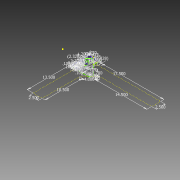
# Autodesk Inventor part: Phone_Holder
Saved by Autodesk Inventor 2013 (Build 170138000, 138)
## iProperties
Created: 2015-03-29
Part Number: Phone_Holder
Material: Generic
Document SubType Name: Modeling
Designer: Pat
Density: 1 g/cm^3
Author: Pat
Autodesk Inventor part; units mm, degrees
ref_plane "YZ Plane" through (0, 0, 0) normal (1, 0, 0) x (0, 1, 0)
ref_plane "XZ Plane" through (0, 0, 0) normal (0, 1, 0) x (-1, 0, 0)
ref_plane "XY Plane" through (0, 0, 0) normal (0, 0, 1) x (1, 0, 0)
sketch "Sketch1" plane through (0, 0, 0) normal (0, 1, 0) x (-1, 0, 0)
  line L0 (-128.4561, -59.0678) -> (-200.4651, -59.0678)
  line L1 (-200.4651, -59.0678) -> (-200.4651, 72.3772)
  line L2 (-200.4651, 72.3772) -> (-128.4561, 72.3772)
  line L3 (-128.4561, 72.3772) -> (-128.4561, 49.0473)
  line L4 (-128.4561, 49.0473) -> (-127.1861, 49.0473)
  line L5 (-127.1861, 49.0473) -> (-127.1861, 38.6333)
  line L6 (-127.1861, 38.6333) -> (-128.4561, 38.6333)
  line L7 (-128.4561, 38.6333) -> (-128.4561, 3.6194)
  line L8 (-128.4561, 3.6194) -> (-127.1861, 3.6194)
  line L9 (-127.1861, 3.6194) -> (-127.1861, -6.7946)
  line L10 (-127.1861, -6.7946) -> (-128.4561, -6.7946)
  line L11 (-128.4561, -6.7946) -> (-128.4561, -20.3074)
  line L12 (-128.4561, -20.3074) -> (-127.1861, -20.3074)
  line L13 (-127.1861, -20.3074) -> (-127.1861, -39.6114)
  line L14 (-127.1861, -39.6114) -> (-128.4561, -39.6114)
  line L15 (-128.4561, -39.6114) -> (-128.4561, -59.0678)
  line L16 (-203.0051, 74.9172) -> (-125.9161, 74.9172)
  line L17 (-125.9161, 74.9172) -> (-125.9161, -61.6078)
  line L18 (-125.9161, -61.6078) -> (-203.0051, -61.6078)
  line L19 (-203.0051, -61.6078) -> (-203.0051, 74.9172)
  circle A0 centre (-164.6511, -28.5878) radius 4.9213 construction
  line L20 (-203.0051, 74.9172) -> (-266.5051, 74.9172)
  line L21 (-164.6511, 373.4543) -> (-228.1511, 373.4543) construction
  line L22 (-228.1511, 373.4543) -> (-228.1511, 106.7543) construction
  line L23 (-228.1511, 106.7543) -> (-299.9932, 34.9122) construction
  line L24 (-299.9932, 34.9122) -> (-668.2932, 34.9122) construction
  line L25 (-668.2932, 34.9122) -> (-668.2932, -28.5878) construction
  line L26 (-668.2932, -28.5878) -> (-223.7932, -28.5878) construction
  line L27 (-223.7932, -28.5878) -> (-164.6511, 30.5543) construction
  line L28 (-164.6511, 30.5543) -> (-164.6511, 373.4543) construction
  line L29 (-264.0722, 70.8332) -> (-194.2222, 0.9832) construction
  line L30 (-164.6511, 30.5543) -> (-164.6511, -28.5878) construction
  line L31 (-164.6511, -28.5878) -> (-223.7932, -28.5878) construction
  circle A1 centre (-251.4998, 58.2609) radius 2.54
  circle A2 centre (-215.5788, 22.3399) radius 1.7653
  line L32 (-266.5051, 74.9172) -> (-266.5051, 49.5172)
  line L33 (-266.5051, 49.5172) -> (-203.0051, -13.9828)
  line L34 (-177.3511, 74.9172) -> (-177.3511, 72.3772)
  line L35 (-151.9511, 74.9172) -> (-151.9511, 72.3772)
  line L36 (-177.3511, -61.6078) -> (-177.3511, -59.0678)
  line L37 (-151.9511, -61.6078) -> (-151.9511, -59.0678)
  line L38 (-266.5051, 68.4003) -> (-259.9882, 74.9172)
  point P0 (0, 0)
  dimension "d0" = 72.009
  dimension "d3" = 131.445
  dimension "d4" = 10.414
  dimension "d5" = 10.414
  dimension "d6" = 19.304
  dimension "d7" = 23.3299
  dimension "d8" = 35.0139
  dimension "d9" = 13.5128
  dimension "d10" = 1.27
  dimension "d11" = 2.54
  dimension "d12" = 2.54
  dimension "d13" = 2.54
  dimension "d14" = 2.54
  dimension "d15" = 9.8425
  dimension "d17" = 36.195
  dimension "d18" = 30.48
  dimension "d19" = 63.5
  dimension "d20" = 63.5
  dimension "d21" = 63.5
  dimension "d22" = 101.6
  dimension "d23" = 266.7
  dimension "d24" = 368.3
  dimension "d25" = 444.5
  dimension "d26" = 342.9
  dimension "d27" = 5.08
  dimension "d28" = 3.5306
  dimension "d29" = 17.78
  dimension "d30" = 68.58
  dimension "d31" = 25.4
  dimension "d44" = 12.7
  dimension "d45" = 12.7
  dimension "d64" = 59.142
  dimension "d65" = 59.142
  constraints: 78 end point, 22 parallel, 15 point on line, 11 perpendicular, 6 collinear, 3 centre point, 2 horizontal, 2 midpoint, 1 coincident
  measures "d0" distance of L0.start L0.end
  measures "d3" distance of L0.end L1.end
  measures "d4" distance of L4.end L5.end
  measures "d5" distance of L8.end L9.end
  measures "d6" distance of L12.end L13.end
  measures "d7" distance of L2.end L3.end
  measures "d8" distance of L6.end L7.end
  measures "d9" distance of L10.end L11.end
  measures "d10" distance of L13.end L14.end
  measures "d11" horizontal distance of L16.end L2.end
  measures "d12" horizontal distance of L1.end L16.start
  measures "d13" horizontal distance of L2.end L16.end
  measures "d14" horizontal distance of L17.end L0.start
  measures "d15" diameter of A0
  measures "d17" horizontal distance of A0.centre L0.start
  measures "d18" vertical distance of L0.start A0.centre
  measures "d19" distance of L16.start L20.end
  measures "d20" distance of L21.start L21.end
  measures "d21" distance of L24.end L25.end
  measures "d22" distance of L22.end L23.end
  measures "d23" distance of L21.end L22.end
  measures "d24" distance of L23.end L24.end
  measures "d25" distance of L25.end L26.end
  measures "d26" distance of L27.end L21.start
  measures "d27" diameter of A1
  measures "d28" diameter of A2
  measures "d29" distance from line of L23 A1.centre
  measures "d30" distance from line of L23 A2.centre
  measures "d31" distance of L20.end L32.end
  measures "d44" distance between parallel lines of L28 L34
  measures "d45" distance between parallel lines of L28 L35
  measures "d64" distance of A0.centre L26.end
  measures "d65" distance of L27.end L30.end
extrude "Extrusion13" add sketch "Sketch1" along normal blind 2.54 contours L0 L1 L2 L3 L4 L5 L6 L7 L8 L9 L10 L11 L12 L13 L14 L15
extrude "Extrusion14" add sketch "Sketch1" along normal blind 3.81 contours L33 L32 L38 L20 L19
extrude "Extrusion15" add sketch "Sketch1" along normal blind 10.16 contours L15 L14 L13 L12 L11 L10 L9 L8 L7 L6 L5 L4 L3 L2 L35 L16 L17 L18 L37 L0 | L36 L18 L19 L16 L34 L2 L1 L0
sketch "Sketch5" plane through (0, 2.54, 0) normal (0, 1, 0) x (1, 0, 0)
  line L0 (200.4651, 59.0678) -> (177.3511, 59.0678) projected
  line L1 (177.3511, 59.0678) -> (151.9511, 59.0678) projected
  line L2 (128.4561, -49.0473) -> (128.4561, -72.3772) projected
  line L3 (128.4561, -72.3772) -> (151.9511, -72.3772) projected
  line L4 (151.9511, -72.3772) -> (177.3511, -72.3772) projected
  line L5 (200.4651, -72.3772) -> (200.4651, 59.0678) projected
  line L6 (151.9511, -72.3772) -> (128.4561, -72.3772) projected
  line L7 (164.6511, 59.0678) -> (164.6511, -72.3772) construction
  line L8 (134.8061, -66.0272) -> (194.1151, -66.0272) construction
  line L9 (194.1151, -66.0272) -> (194.1151, 52.7178) construction
  line L10 (194.1151, 52.7178) -> (134.8061, 52.7178) construction
  line L11 (134.8061, 52.7178) -> (134.8061, -66.0272) construction
  line L12 (134.8061, -66.0272) -> (153.8561, -66.0272)
  line L13 (153.8561, -66.0272) -> (134.8061, -46.9772)
  line L14 (134.8061, -46.9772) -> (134.8061, -66.0272)
  line L15 (194.1151, -66.0272) -> (175.0651, -66.0272)
  line L16 (175.0651, -66.0272) -> (194.1151, -46.9772)
  line L17 (194.1151, -46.9772) -> (194.1151, -66.0272)
  line L18 (164.6511, -66.0272) -> (162.1111, -66.0272)
  line L19 (162.1111, -66.0272) -> (134.8061, -38.7222)
  line L20 (134.8061, -38.7222) -> (134.8061, -31.1022)
  line L21 (134.8061, -31.1022) -> (162.7461, -59.0422)
  line L22 (162.7461, -59.0422) -> (166.5561, -59.0422)
  line L23 (166.5561, -59.0422) -> (194.1151, -31.4832)
  line L24 (194.1151, -31.4832) -> (194.1151, -39.1032)
  line L25 (194.1151, -39.1032) -> (167.1911, -66.0272)
  line L26 (167.1911, -66.0272) -> (164.6511, -66.0272)
  line L27 (194.1151, -6.6547) -> (134.8061, -6.6547) construction
  line L28 (164.6511, -20.3333) -> (157.5713, -10.4647)
  line L29 (157.5713, -10.4647) -> (146.6493, -10.4647)
  line L30 (146.6493, -10.4647) -> (146.6493, -18.0847)
  line L31 (146.6493, -18.0847) -> (149.1893, -18.0847)
  line L32 (149.1893, -18.0847) -> (149.1893, -30.0227)
  line L33 (149.1893, -30.0227) -> (146.6493, -30.0227)
  line L34 (146.6493, -30.0227) -> (146.6493, -37.6427)
  line L35 (146.6493, -37.6427) -> (160.6193, -37.6427)
  line L36 (160.6193, -37.6427) -> (160.6193, -30.0227)
  line L37 (160.6193, -30.0227) -> (157.3173, -30.0227)
  line L38 (157.3173, -30.0227) -> (157.3173, -22.4027)
  line L39 (157.3173, -22.4027) -> (164.6511, -32.6253)
  line L40 (164.6511, -20.3333) -> (171.731, -10.4647)
  line L41 (171.731, -10.4647) -> (182.653, -10.4647)
  line L42 (182.653, -10.4647) -> (182.653, -18.0847)
  line L43 (182.653, -18.0847) -> (180.113, -18.0847)
  line L44 (180.113, -18.0847) -> (180.113, -30.0227)
  line L45 (180.113, -30.0227) -> (182.653, -30.0227)
  line L46 (182.653, -30.0227) -> (182.653, -37.6427)
  line L47 (182.653, -37.6427) -> (168.683, -37.6427)
  line L48 (168.683, -37.6427) -> (168.683, -30.0227)
  line L49 (168.683, -30.0227) -> (171.985, -30.0227)
  line L50 (171.985, -30.0227) -> (171.985, -22.4027)
  line L51 (171.985, -22.4027) -> (164.6511, -32.6253)
  line L52 (154.6041, -43.9927) -> (182.6357, -43.9927) construction
  line L53 (182.6357, -43.9927) -> (182.6357, -47.2383) construction
  line L54 (182.6357, -47.2383) -> (154.6041, -47.2383) construction
  line L55 (154.6041, -47.2383) -> (154.6041, -43.9927) construction
  line L56 (134.8061, 52.7178) -> (194.1151, 52.7178) construction
  line L57 (134.8061, 52.7178) -> (153.8561, 52.7178)
  line L58 (153.8561, 52.7178) -> (134.8061, 33.6678)
  line L59 (134.8061, 33.6678) -> (134.8061, 52.7178)
  line L60 (194.1151, 52.7178) -> (175.0651, 52.7178)
  line L61 (175.0651, 52.7178) -> (194.1151, 33.6678)
  line L62 (194.1151, 33.6678) -> (194.1151, 52.7178)
  line L63 (164.6511, 52.7178) -> (162.1111, 52.7178)
  line L64 (162.1111, 52.7178) -> (134.8061, 25.4128)
  line L65 (134.8061, 25.4128) -> (134.8061, 17.7928)
  line L66 (134.8061, 17.7928) -> (162.7461, 45.7328)
  line L67 (162.7461, 45.7328) -> (166.5561, 45.7328)
  line L68 (166.5561, 45.7328) -> (194.1151, 18.1738)
  line L69 (194.1151, 18.1738) -> (194.1151, 25.7938)
  line L70 (194.1151, 25.7938) -> (167.1911, 52.7178)
  line L71 (167.1911, 52.7178) -> (164.6511, 52.7178)
  line L72 (164.6511, 7.0239) -> (157.5713, -2.8447)
  line L73 (157.5713, -2.8447) -> (146.6493, -2.8447)
  line L74 (146.6493, -2.8447) -> (146.6493, 4.7753)
  line L75 (146.6493, 4.7753) -> (149.1893, 4.7753)
  line L76 (149.1893, 4.7753) -> (149.1893, 16.7133)
  line L77 (149.1893, 16.7133) -> (146.6493, 16.7133)
  line L78 (146.6493, 16.7133) -> (146.6493, 24.3333)
  line L79 (146.6493, 24.3333) -> (160.6193, 24.3333)
  line L80 (160.6193, 24.3333) -> (160.6193, 16.7133)
  line L81 (160.6193, 16.7133) -> (157.3173, 16.7133)
  line L82 (157.3173, 16.7133) -> (157.3173, 9.0933)
  line L83 (157.3173, 9.0933) -> (164.6511, 19.3159)
  line L84 (180.113, 16.7133) -> (182.653, 16.7133)
  line L85 (168.683, 24.3333) -> (168.683, 16.7133)
  line L86 (182.653, 16.7133) -> (182.653, 24.3333)
  line L87 (168.683, 16.7133) -> (171.985, 16.7133)
  line L88 (182.653, 24.3333) -> (168.683, 24.3333)
  line L89 (171.985, 9.0933) -> (164.6511, 19.3159)
  line L90 (171.985, 16.7133) -> (171.985, 9.0933)
  line L91 (180.113, 4.7753) -> (180.113, 16.7133)
  line L92 (182.653, 4.7753) -> (180.113, 4.7753)
  line L93 (164.6511, 7.0239) -> (171.731, -2.8447)
  line L94 (171.731, -2.8447) -> (182.653, -2.8447)
  line L95 (182.653, -2.8447) -> (182.653, 4.7753)
  line L96 (174.6875, 30.6833) -> (147.7056, 30.6833) construction
  line L97 (147.7056, 30.6833) -> (147.7056, 39.0913) construction
  line L98 (147.7056, 39.0913) -> (174.6875, 39.0913) construction
  line L99 (174.6875, 39.0913) -> (174.6875, 30.6833) construction
  point P0 (0, 0)
  dimension "d78" = 6.35
  dimension "d79" = 6.35
  dimension "d80" = 6.35
  dimension "d81" = 6.35
  dimension "d82" = 19.05
  dimension "d83" = 45
  dimension "d84" = 19.05
  dimension "d85" = 45
  dimension "d87" = 135
  dimension "d88" = 7.62
  dimension "d89" = 45
  dimension "d90" = 3.81
  dimension "d91" = 135
  dimension "d92" = 7.62
  dimension "d93" = 135
  dimension "d94" = 5.08
  dimension "d95" = 13.97
  dimension "d96" = 7.62
  dimension "d97" = 8.128
  dimension "d98" = 11.938
  dimension "d99" = 2.54
  dimension "d100" = 7.62
  dimension "d101" = 10.922
  dimension "d102" = 7.62
  dimension "d103" = 3.81
  dimension "d104" = 6.35
  dimension "d105" = 6.35
  constraints: 170 end point, 48 symmetric about line, 19 point on line, 12 perpendicular, 6 parallel, 4 midpoint, 3 collinear, 4 other
  measures "d78" distance between parallel lines of L8 L3
  measures "d79" distance between parallel lines of L2 L11
  measures "d80" distance between parallel lines of L9 L5
  measures "d81" distance between parallel lines of L0 L10
  measures "d82" distance of L8.start L12.end
  measures "d83" angle of L13 L12
  measures "d84" distance of L8.end L15.end
  measures "d85" angle of L15 L16
  measures "d87" angle of L18 L19
  measures "d88" distance of L19.end L20.end
  measures "d89" angle of L20 L21
  measures "d90" distance of L21.end L22.end
  measures "d91" angle of L23 L22
  measures "d92" distance of L23.end L24.end
  measures "d93" angle of L24 L25
  measures "d94" distance of L25.end L18.end
  measures "d95" distance of L34.end L35.end
  measures "d96" distance of L33.end L34.end
  measures "d97" distance of L37.end L32.end
  measures "d98" distance of L31.end L32.end
  measures "d99" distance of L30.end L31.end
  measures "d100" distance of L29.end L30.end
  measures "d101" distance of L28.end L29.end
  measures "d102" distance of L37.end L38.end
  measures "d103" distance between parallel lines of L27 L29
  measures "d104" distance between parallel lines of L35 L52
  measures "d105" distance between parallel lines of L88 L96
extrude "Extrusion16" cut sketch "Sketch5" against normal blind 25.4
sketch "Sketch6" plane through (0, 3.81, 0) normal (0, 1, 0) x (1, 0, 0)
  circle A0 centre (251.4998, -58.2609) radius 2.54 projected
  circle A1 centre (215.5788, -22.3399) radius 1.7653 projected
  line L0 (203.0051, -74.9172) -> (259.9882, -74.9172) projected
  line L1 (259.9882, -74.9172) -> (266.5051, -68.4003) projected
  line L2 (266.5051, -68.4003) -> (266.5051, -49.5172) projected
  line L3 (266.5051, -49.5172) -> (203.0051, 13.9828) projected
  line L4 (203.0051, 13.9828) -> (203.0051, -74.9172) projected
  line L5 (205.5451, -68.5672) -> (257.3579, -68.5672) construction
  line L6 (257.3579, -68.5672) -> (260.1551, -65.77) construction
  line L7 (260.1551, -65.77) -> (260.1551, -52.1475) construction
  line L8 (260.1551, -52.1475) -> (205.5451, 2.4625) construction
  line L9 (205.5451, 2.4625) -> (205.5451, -68.5672) construction
  line L10 (245.7848, -68.5672) -> (245.7848, -53.3272)
  line L11 (245.7848, -53.3272) -> (253.5598, -45.5522)
  line L12 (249.5187, -41.5111) -> (240.0698, -50.96)
  line L13 (240.0698, -50.96) -> (240.0698, -68.5672)
  line L14 (240.0698, -68.5672) -> (245.7848, -68.5672)
  line L15 (253.5598, -45.5522) -> (249.5187, -41.5111)
  line L16 (234.9898, -68.5672) -> (234.9898, -48.8558)
  line L17 (234.9898, -48.8558) -> (245.9266, -37.919)
  line L18 (241.8855, -33.8778) -> (229.2748, -46.4885)
  line L19 (229.2748, -46.4885) -> (229.2748, -68.5672)
  line L20 (234.9898, -68.5672) -> (229.2748, -68.5672)
  line L21 (245.9266, -37.919) -> (241.8855, -33.8778)
  line L22 (224.1948, -68.5672) -> (224.1948, -44.3843)
  line L23 (224.1948, -44.3843) -> (238.2934, -30.2857)
  line L24 (218.4798, -68.5672) -> (218.4798, -42.0171)
  line L25 (218.4798, -42.0171) -> (234.2523, -26.2446)
  line L26 (234.2523, -26.2446) -> (238.2934, -30.2857)
  line L27 (224.1948, -68.5672) -> (218.4798, -68.5672)
  line L28 (230.6602, -22.6525) -> (213.3998, -39.9129)
  line L29 (213.3998, -39.9129) -> (213.3998, -68.5672)
  line L30 (207.6848, -68.5672) -> (207.6848, -37.5457)
  line L31 (207.6848, -37.5457) -> (226.6191, -18.6114)
  line L32 (226.6191, -18.6114) -> (230.6602, -22.6525)
  line L33 (207.6848, -68.5672) -> (213.3998, -68.5672)
  line L34 (207.6848, -23.2472) -> (210.6385, -20.2935)
  line L35 (210.6385, -20.2935) -> (210.6385, -20.2935)
  line L36 (210.6385, -20.2935) -> (219.4698, -11.4622)
  line L37 (207.6848, -23.2472) -> (207.6848, -15.165)
  line L38 (207.6848, -15.165) -> (215.4287, -7.421)
  line L39 (215.4287, -7.421) -> (219.4698, -11.4622)
  line L40 (211.8366, -3.8289) -> (207.6848, -7.9808)
  line L41 (207.6848, -7.9808) -> (207.6848, 0.3229)
  line L42 (211.8366, -3.8289) -> (207.6848, 0.3229)
  point P0 (0, 0)
  dimension "d108" = 6.35
  dimension "d109" = 6.35
  dimension "d110" = 6.35
  dimension "d111" = 6.35
  dimension "d112" = 2.54
  dimension "d113" = 15.24
  dimension "d114" = 3.175
  dimension "d115" = 5.715
  dimension "d116" = 5.715
  dimension "d117" = 5.08
  dimension "d118" = 5.715
  dimension "d119" = 5.715
  dimension "d120" = 5.08
  dimension "d121" = 5.08
  dimension "d122" = 5.08
  dimension "d123" = 5.715
  dimension "d124" = 5.715
  dimension "d127" = 5.08
  dimension "d128" = 5.715
  dimension "d129" = 5.715
  dimension "d130" = 5.08
  dimension "d131" = 3.405
  dimension "d132" = 4.9897
  dimension "d133" = 5.715
  dimension "d134" = 3.175
  dimension "d136" = 3.175
  dimension "d137" = 5.08
  constraints: 72 end point, 8 perpendicular, 6 parallel, 5 collinear, 5 vertical, 4 horizontal, 36 other
  measures "d109" distance between parallel lines of L6 L1
  measures "d110" distance between parallel lines of L2 L7
  measures "d112" distance between parallel lines of L4 L9
  measures "d113" distance of L10.start L10.end
  measures "d114" distance edge to line of A0 L10
  measures "d115" distance between parallel lines of L13 L10
  measures "d116" distance between parallel lines of L12 L11
  measures "d117" distance between parallel lines of L13 L16
  measures "d118" distance between parallel lines of L19 L16
  measures "d119" distance between parallel lines of L18 L17
  measures "d120" distance between parallel lines of L17 L12
  measures "d121" distance between parallel lines of L19 L22
  measures "d122" distance between parallel lines of L23 L18
  measures "d123" distance between parallel lines of L22 L24
  measures "d124" distance between parallel lines of L25 L23
  measures "d127" distance between parallel lines of L28 L25
  measures "d128" distance between parallel lines of L31 L28
  measures "d129" distance between parallel lines of L30 L29
  measures "d130" distance between parallel lines of L29 L24
  measures "d131" distance edge to line of A1 L31
  measures "d132" distance edge to line of A0 L11
  measures "d133" distance between parallel lines of L38 L36
  measures "d134" distance edge to line of A1 L36
  measures "d136" distance edge to line of A1 L35
  measures "d137" distance between parallel lines of L40 L38
extrude "Extrusion17" cut sketch "Sketch6" against normal blind 12.7 contours L14 L13 L12 L15 L11 L10 | L20 L19 L18 L21 L17 L16 | L27 L24 L25 L26 L23 L22 | L28 L29 L33 L30 L31 L32 | L37 L38 L39 L36 L34 | L40 L41 L42
body "Solid5"
